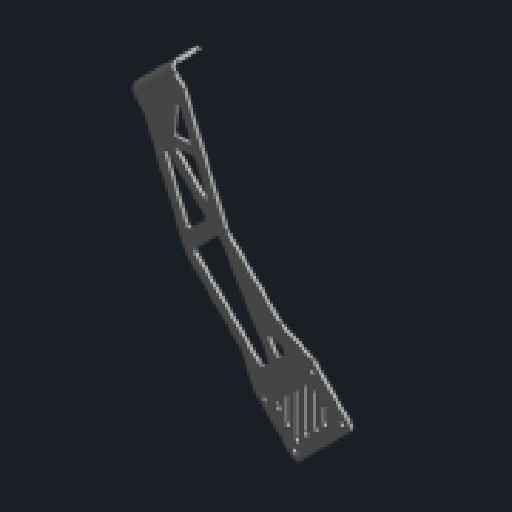
# Autodesk Inventor part: ArmScapula
Saved by Autodesk Inventor 2025.2 (Build 292293000, 293)
## iProperties
Created: 2025-02-16
Part Number: ArmScapula
Material: Generic
Document SubType Name: Sheet Metal
Designer: valer
Density: 1 g/cm^3
Appearance: Default
Sheet Metal Rule: Default
Author: valer
Autodesk Inventor part; units mm, degrees
ref_plane "YZ Plane" through (0, 0, 0) normal (1, 0, 0) x (0, 1, 0)
ref_plane "XZ Plane" through (0, 0, 0) normal (0, 1, 0) x (-1, 0, 0)
ref_plane "XY Plane" through (0, 0, 0) normal (0, 0, 1) x (1, 0, 0)
sketch "Base" plane through (0, 0, 0) normal (0, 0, 1) x (1, 0, 0)
  line L0 (-51.7107, 91.7107) -> (-70.8448, 137.9047)
  line L1 (-110.8448, 137.9047) -> (-79.9949, 63.4264)
  line L2 (-79.9949, 63.4264) -> (-23, 6.4315)
  line L3 (-51.7107, 91.7107) -> (-79.9949, 63.4264) construction
  line L4 (-23.574, 44.8219) -> (-5.7487, 37.2635)
  line L5 (-5.7487, 37.2635) -> (-14.0998, 28.9124)
  line L6 (-14.0998, 28.9124) -> (-23.574, 44.8219)
  line L7 (-55.9533, 87.468) -> (-75.7523, 67.669)
  line L8 (-75.7523, 67.669) -> (-25.5477, 17.4645)
  line L9 (-61.2778, 114.8077) -> (-95.4199, 100.6655) construction
  line L10 (-55.9533, 87.468) -> (-18.4767, 24.5355)
  line L11 (-18.4767, 24.5355) -> (-25.5477, 17.4645)
  line L12 (-73.1971, 127.9047) -> (-60.445, 97.1185)
  line L13 (-60.445, 97.1185) -> (-79.5449, 78.0186)
  line L14 (-79.5449, 78.0186) -> (-100.2084, 127.9047)
  line L15 (-100.2084, 127.9047) -> (-73.1971, 127.9047)
  line L16 (-14.0998, 28.9124) -> (-18.4767, 24.5355) construction
  line L17 (-51.7107, 91.7107) -> (5.2843, 34.7157)
  line L18 (-64.6877, 92.8758) -> (-100.5562, 128.7444)
  line L19 (-60.445, 97.1185) -> (-91.2312, 127.9047)
  line L20 (-70.8448, 137.9047) -> (-110.8448, 137.9047)
  line L21 (-23, 6.4315) -> (5.2843, 34.7157)
  point P0 (0, 0)
  point P1 (-66.821, 112.5116)
  point P2 (-51.4975, 34.9289)
  point P3 (-99.7165, 127.9047)
  dimension "d4" = 6
  dimension "d7" = 6
  dimension "d8" = 6
  dimension "d9" = 6
  dimension "d22" = 10
  dimension "d23" = 6
  dimension "d29" = 50
  dimension "d30" = 10
  dimension "d79" = 6
  dimension "d124" = 67.978
  dimension "d125" = 6
  measures "d4" distance from line of point (-51.497, 34.929) L8
  measures "d7" distance of L0.start L7.start
  measures "d8" distance between parallel lines of L1 L14
  measures "d9" distance between parallel lines of L0 L12
  measures "d22" distance between parallel lines of L7 L13
  measures "d23" distance from line of L17 L4.end
  measures "d29" distance of L0.start L0.end
  measures "d30" distance of L10.end L8.end
  measures "d79" distance between parallel lines of L18 L19
  measures "d124" angle of L5 L4
  measures "d125" distance between parallel lines of L10 L6
extrude "Plate1" add sketch "Base" along normal blind 3.048 contours L17 L21 L2 L1 L20 L0 | L13 L18 L15 L19
delete faces "Delete1" heal yes whole lump no faces at (-100.0444, 127.9047, 1.016)
fillet "InsideFilletsFeature" radius 2 13 edges at (-5.7487, 37.2635, 1.524) (-14.0998, 28.9124, 1.524) (-23.574, 44.8219, 1.524) (-25.5477, 17.4645, 1.524) (-18.4767, 24.5355, 1.524) (-55.9533, 87.468, 1.524) (-75.7523, 67.669, 1.524) (-79.5449, 78.0186, 1.524) (-60.445, 97.1185, 1.524) (-73.1971, 127.9047, 1.524) (-64.6877, 92.8758, 1.524) (-91.2312, 127.9047, 1.524) (-100.5562, 128.7444, 1.524)
sketch "Mount" plane through (-70.8448, 137.9047, 0) normal (0, 0, -1) x (-1, 0, 0)
  arc A0 (-84.819, -103.9794) -> (-83.1169, -102.2772) centre (-83.2002, -103.896) ccw construction
  arc A1 (-106.7394, -125.8997) -> (-105.0372, -124.1975) centre (-105.1205, -125.8163) ccw construction
  arc A2 (-46.9331, -138.4609) -> (-48.6353, -140.1631) centre (-48.552, -138.5443) ccw construction
  arc A3 (-68.8534, -160.3813) -> (-70.5556, -162.0834) centre (-70.4723, -160.4646) ccw construction
  line L0 (-47.8448, -131.4732) -> (-76.1291, -103.1889)
  line L1 (-47.8448, -131.4732) -> (9.1501, -74.4782)
  line L2 (-30.929, -114.5574) -> (-41.688, -137.6301)
  line L3 (-41.688, -137.6301) -> (-71.3865, -167.3285)
  line L4 (-71.3865, -167.3285) -> (-112.1916, -126.5234)
  line L5 (-112.1916, -126.5234) -> (-82.4931, -96.825)
  line L6 (-82.4931, -96.825) -> (-58.6443, -85.7041)
  line L7 (-76.1291, -103.1889) -> (-19.1342, -46.194)
  line L8 (-44.1022, -138.6301) -> (-70.3865, -164.9143) construction
  line L9 (-83.4931, -99.2392) -> (-109.7774, -125.5234) construction
  line L10 (-109.7774, -128.9377) -> (-73.5936, -165.1214) construction
  circle A4 centre (-48.552, -138.5443) radius 2
  circle A5 centre (-70.4723, -160.4646) radius 2
  circle A6 centre (-83.2002, -103.896) radius 2
  circle A7 centre (-105.1205, -125.8163) radius 2
  point P0 (-70.8448, -137.9047)
sheet face with bend "MountFeature" sketch "Mount" thickness 3.048 toward (0, 0, 1) bend radius 3.048 relief straight relief width 3.048 relief depth 1.524
bend "Bend4"
fillet "OutsideFilletsFeature" radius 4 8 edges at (0.5416, -29.4239, 1.524) (41.3467, 11.3812, 1.524) (11.6482, 41.0797, 1.524) (-29.1569, 0.2746, 1.524) (-39.9158, 23.3473, 1.524) (-12.2006, 52.2006, 1.524) (-79.9949, 63.4264, 1.524) (-51.7107, 91.7107, 1.524)
sketch "VentHoles" plane through (-70.8448, 137.9047, 0) normal (0, 0, -1) x (-1, 0, 0)
  line L0 (-58.536, -135.9217) -> (-58.536, -138.9217) construction
  line L1 (-60.536, -135.9217) -> (-60.536, -138.9217)
  line L2 (-56.536, -138.9217) -> (-56.536, -135.9217)
  arc A0 (-56.536, -135.9217) -> (-60.536, -135.9217) centre (-58.536, -135.9217) ccw
  arc A1 (-60.536, -138.9217) -> (-56.536, -138.9217) centre (-58.536, -138.9217) ccw
  circle A2 centre (-48.552, -138.5443) radius 2 construction
  circle A3 centre (-105.1205, -125.8163) radius 2 construction
  line L3 (-65.3148, -145.7005) -> (-65.3148, -129.1429) construction
  line L4 (-63.3148, -145.7005) -> (-63.3148, -129.1429)
  line L5 (-67.3148, -129.1429) -> (-67.3148, -145.7005)
  arc A4 (-67.3148, -145.7005) -> (-63.3148, -145.7005) centre (-65.3148, -145.7005) ccw
  arc A5 (-63.3148, -129.1429) -> (-67.3148, -129.1429) centre (-65.3148, -129.1429) ccw
  line L6 (-72.0936, -122.3641) -> (-72.0936, -152.4793) construction
  line L7 (-74.0936, -122.3641) -> (-74.0936, -152.4793)
  line L8 (-70.0936, -152.4793) -> (-70.0936, -122.3641)
  arc A6 (-70.0936, -122.3641) -> (-74.0936, -122.3641) centre (-72.0936, -122.3641) ccw
  arc A7 (-74.0936, -152.4793) -> (-70.0936, -152.4793) centre (-72.0936, -152.4793) ccw
  circle A8 centre (-70.4723, -160.4646) radius 2 construction
  line L9 (-78.8724, -115.5852) -> (-78.8724, -145.7005) construction
  line L10 (-76.8724, -115.5852) -> (-76.8724, -145.7005)
  line L11 (-80.8724, -145.7005) -> (-80.8724, -115.5852)
  arc A9 (-76.8724, -115.5852) -> (-80.8724, -115.5852) centre (-78.8724, -115.5852) ccw
  arc A10 (-80.8724, -145.7005) -> (-76.8724, -145.7005) centre (-78.8724, -145.7005) ccw
  line L12 (-85.6512, -115.5394) -> (-85.6512, -138.9217) construction
  line L13 (-87.6512, -115.5394) -> (-87.6512, -138.9217)
  line L14 (-83.6512, -138.9217) -> (-83.6512, -115.5394)
  arc A11 (-83.6512, -115.5394) -> (-87.6512, -115.5394) centre (-85.6512, -115.5394) ccw
  arc A12 (-87.6512, -138.9217) -> (-83.6512, -138.9217) centre (-85.6512, -138.9217) ccw
  circle A13 centre (-83.2002, -103.896) radius 2 construction
  line L15 (-92.43, -132.1429) -> (-92.43, -122.3183) construction
  line L16 (-94.43, -132.1429) -> (-94.43, -122.3183)
  line L17 (-90.43, -122.3183) -> (-90.43, -132.1429)
  arc A14 (-94.43, -132.1429) -> (-90.43, -132.1429) centre (-92.43, -132.1429) ccw
  arc A15 (-90.43, -122.3183) -> (-94.43, -122.3183) centre (-92.43, -122.3183) ccw
  line L18 (-54.2075, -137.4217) -> (-72.0936, -155.3077) construction
  line L19 (-72.0936, -155.3077) -> (-100.1708, -127.2306) construction
  line L20 (-100.1708, -127.2306) -> (-82.2847, -109.3445) construction
  line L21 (-82.2847, -109.3445) -> (-54.2075, -137.4217) construction
  line L22 (-46.7113, -119.026) -> (-51.2678, -114.4695) construction
  line L23 (-68.5581, -164.5001) -> (-42.1867, -138.1288) construction
  line L24 (-109.3631, -129.3519) -> (-74.2149, -164.5001) construction
  line L25 (-82.9918, -97.3237) -> (-109.3631, -123.695) construction
  point P0 (-70.8448, -137.9047)
  point P1 (-58.536, -137.4217)
  point P2 (-65.3148, -137.4217)
  point P3 (-72.0936, -137.4217)
  point P4 (-78.8724, -130.6429)
  point P5 (-85.6512, -127.2306)
  point P6 (-92.43, -127.2306)
  point P7 (-97.6499, -127.9377)
  dimension "d142" = 4
  dimension "d158" = 6.7788
  dimension "d159" = 6.7788
  dimension "d160" = 6.7788
  dimension "d161" = 6.7788
  dimension "d162" = 6.7788
  dimension "d164" = 9
  dimension "d165" = 8
  dimension "d166" = 9
  dimension "d167" = 8
  dimension "d168" = 45
  dimension "d170" = 3
  constraints: 56 end point, 37 tangent, 24 point on circle, 12 centre point, 12 parallel, 6 midpoint, 5 equal radius, 2 perpendicular
  measures "d142" diameter of A1
  measures "d158" distance between parallel lines of L3 L0
  measures "d159" distance between parallel lines of L6 L3
  measures "d160" distance between parallel lines of L9 L6
  measures "d161" distance between parallel lines of L12 L9
  measures "d162" distance between parallel lines of L15 L12
  measures "d164" distance between parallel lines of L23 L18
  measures "d165" distance between parallel lines of L24 L19
  measures "d166" distance between parallel lines of L25 L20
  measures "d167" distance from line of L23.end L21
  measures "d168" angle of L21 L0
  measures "d170" distance of L0.start L0.end
extrude "VentHolesFeature" cut sketch "VentHoles" against normal blind 3.048
sketch "Connector" plane through (-70.8448, 137.9047, 0) normal (0, 0, -1) x (-1, 0, 0)
  line L0 (40, 0) -> (9.4546, -73.7432)
  line L1 (-18.8297, -45.4589) -> (0, 0)
  line L2 (40, 0) -> (0, 0)
  line L3 (0, 0) -> (11.7157, 28.2843)
  line L4 (11.7157, 28.2843) -> (23.0294, 39.598)
  line L5 (23.0294, 39.598) -> (51.3137, 11.3137)
  line L6 (51.3137, 11.3137) -> (40, 0)
  line L7 (40, 0) -> (11.7157, 28.2843) construction
  line L8 (-68.5581, -164.5001) -> (-42.1867, -138.1288)
  point P0 (-70.8448, -137.9047)
  point P1 (25.8579, 14.1421)
  point P2 (20, 0)
  dimension "d177" = 16
  measures "d177" distance of L5.end L0.start
sheet face with bend "ConnectorFeature" sketch "Connector" thickness 3.048 toward (0, 0, 1) bend radius 3.048 relief straight relief width 3.048 relief depth 1.524
bend "Bend5"
sketch "Sketch18" plane through (-91.719, 175.3474, 3.048) normal (-0.7071068, 0.7071068, 0) x (-0.7071068, -0.7071068, 0)
  line L0 (40, 0) -> (0, 0)
  line L1 (0, 0) -> (0, -25)
  line L2 (0, -25) -> (40, -25)
  line L3 (40, -25) -> (40, 0)
  constraints: 6 end point, 1 horizontal, 1 perpendicular, 1 vertical
edge flange "BodyMountFeature" height 25 angle 90 thickness 3.048 bend radius 3.048 thickness toward (-0.7071068, 0.7071068, 0) relief straight relief width 3.048 relief depth 1.524 edges at (-108.0164, 163.3605, 0) wall of the first edge with corners at (-120.0033, 147.0631, 3.048) (-91.719, 175.3474, 3.048) (-91.719, 175.3474, -21.952) (-120.0033, 147.0631, -21.952)
bend "Bend6"
corner "Corner4"
fillet "BodyMountFilletsFeature" radius 4 2 edges at (-121.0809, 148.1407, -21.952) (-92.7967, 176.425, -21.952)
sketch "Sketch19" plane through (0.5416, -23.767, 0) normal (0, 0, -1) x (-1, 0, 0)
  line L0 (90.4405, 156.9373) -> (75.9198, 156.9373)
  line L1 (75.9198, 156.9373) -> (87.6944, 185.3638)
  line L2 (87.6944, 185.3638) -> (90.4405, 156.9373)
  line L3 (83.1022, 189.956) -> (52.5568, 116.2128) projected
  line L4 (111.3865, 161.6717) -> (83.1022, 189.956)
  line L5 (64.8344, 130.1748) -> (73.2273, 150.437) construction
  line L6 (75.0751, 151.6717) -> (86.9444, 151.6717) construction
  point P0 (0.5416, 23.767)
  constraints: 8 end point, 1 collinear, 1 parallel, 1 point on line
extrude "BodyMountCutFeature" cut sketch "Sketch19" against normal blind 3.048
fillet "BodyMountInsideFilletsFeature" radius 2 3 edges at (-89.8988, 133.1703, 1.524) (-75.3782, 133.1703, 1.524) (-87.1528, 161.5967, 1.524)
sketch "Sketch20" plane through (-122.1586, 149.2184, -17.952) normal (-0.7071068, 0.7071068, 0) x (-0.7071068, -0.7071068, 0)
  line L0 (-8, 5) -> (-32, 5) construction
  line L1 (-4, -4) -> (-36, -4) construction
  line L2 (0, 14.904) -> (0, 0) construction
  line L3 (-40, 0) -> (-40, 14.904) construction
  circle A0 centre (-8, 5) radius 3
  circle A1 centre (-32, 5) radius 3
  point P0 (19.1342, 17.952)
  dimension "d192" = 8
  dimension "d193" = 8
  dimension "d194" = 9
  dimension "d195" = 6
  constraints: 2 centre point, 2 coincident, 2 end point, 1 equal radius, 1 parallel
  measures "d192" distance from line of L2 L0.start
  measures "d193" distance from line of L3 L0.end
  measures "d194" distance between parallel lines of L1 L0
  measures "d195" diameter of A0
extrude "BodyMountHolesFeature" cut sketch "Sketch20" against normal blind 3.048
equation "\"d22\" = 2 * d3"
equation "\"d3\" = 5"
body "Solid2"
